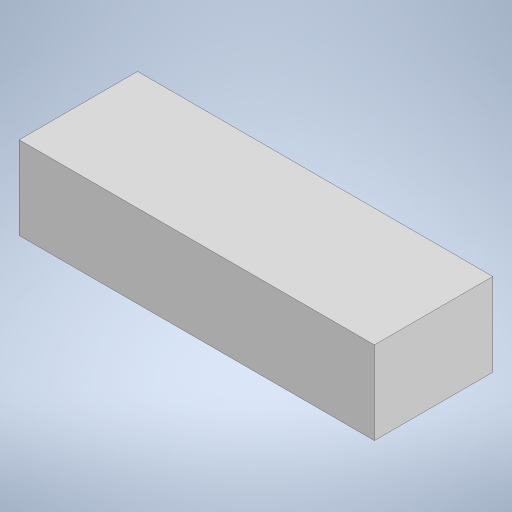
# Autodesk Inventor part: Battery for UAV
Saved by Autodesk Inventor 2023 (Build 270158000, 158)
## iProperties
Created: 2023-02-27
Part Number: Battery for UAV
Material: Generic
Document SubType Name: Modeling
Designer: mihal
Density: 1 g/cm^3
Appearance: Default
Author: mihal
Autodesk Inventor part; units mm, degrees
ref_plane "YZ Plane" through (0, 0, 0) normal (1, 0, 0) x (0, 1, 0)
ref_plane "XZ Plane" through (0, 0, 0) normal (0, 1, 0) x (-1, 0, 0)
ref_plane "XY Plane" through (0, 0, 0) normal (0, 0, 1) x (1, 0, 0)
sketch "Sketch1" plane through (0, 0, 0) normal (0, 1, 0) x (-1, 0, 0)
  line L0 (-75, 25) -> (75, 25)
  line L1 (75, 25) -> (75, -25)
  line L2 (75, -25) -> (-75, -25)
  line L3 (-75, -25) -> (-75, 25)
  line L4 (-75, 25) -> (75, -25) construction
  line L5 (75, 25) -> (-75, -25) construction
  point P0 (0, 0)
  dimension "d0" = 150
  dimension "d1" = 50
  constraints: 12 end point, 2 midpoint, 2 parallel, 1 horizontal, 1 perpendicular
  measures "d0" distance of L1.end L2.end
  measures "d1" distance of L0.end L1.end
extrude "Extrusion1" add sketch "Sketch1" along normal blind 35
body "Solid1"
